Autodesk Fusion 360 part; units mm, degrees
(part 2 of 2)
  spline S394 degree 3 poles (31.1486, 13.7412) (31.2093, 13.8706) (31.3161, 13.9767) (31.4461, 14.036) knots 0.000003 0.000003 0.000003 0.000003 1 1 1 1
  spline S395 degree 3 poles (31.4461, 14.036) (31.5723, 14.0937) (31.7158, 14.1162) (31.8763, 14.1162) knots 0 0 0 0 1 1 1 1
  line L154 (31.8763, 14.1162) -> (34.2237, 14.1162)
  spline S396 degree 3 poles (34.2237, 14.1162) (34.412, 14.1162) (34.5847, 14.0747) (34.7123, 13.9582) knots 0 0 0 0 1 1 1 1
  spline S397 degree 3 poles (34.7123, 13.9582) (34.8291, 13.8516) (34.8932, 13.693) (34.8932, 13.5339) knots 0 0 0 0 1 1 1 1
  spline S398 degree 3 poles (34.8932, 13.5339) (34.8932, 13.3734) (34.8299, 13.2135) (34.7123, 13.1062) knots 0 0 0 0 1 1 1 1
  spline S399 degree 3 poles (34.7123, 13.1062) (34.5847, 12.9897) (34.412, 12.9482) (34.2237, 12.9482) knots 0 0 0 0 1 1 1 1
  line L155 (34.2237, 12.9482) -> (32.4619, 12.9482)
  line L156 (32.4619, 12.9482) -> (32.4619, 12.0907)
  line L157 (32.4619, 12.0907) -> (33.9017, 12.0907)
  spline S400 degree 3 poles (33.9017, 12.0907) (34.0837, 12.0907) (34.2521, 12.0498) (34.3768, 11.9363) knots 0 0 0 0 1 1 1 1
  spline S401 degree 3 poles (34.3768, 11.9363) (34.4927, 11.8307) (34.5545, 11.6729) (34.5545, 11.5151) knots 0 0 0 0 1 1 1 1
  spline S402 degree 3 poles (34.5545, 11.5151) (34.5545, 11.3566) (34.4909, 11.1978) (34.3728, 11.0935) knots 0 0 0 0 1 1 1 1
  spline S403 degree 3 poles (34.3728, 11.0935) (34.2479, 10.9833) (34.0814, 10.9429) (33.9017, 10.9429) knots 0 0 0 0 1 1 1 1
  line L158 (33.9017, 10.9429) -> (32.4619, 10.9429)
  line L159 (32.4619, 10.9429) -> (32.4619, 9.5231)
  spline S404 degree 3 poles (32.4619, 9.5231) (32.4619, 9.2874) (32.4087, 9.0787) (32.269, 8.929) knots 0 0 0 0 1 1 1 1
  spline S405 degree 3 poles (35.2745, 13.3964) (35.2745, 13.628) (35.3278, 13.8341) (35.4642, 13.9838) knots 0 0 0 0 1 1 1 1
  spline S406 degree 3 poles (35.4642, 13.9838) (35.5913, 14.1233) (35.776, 14.2) (35.9675, 14.2) knots 0 0 0 0 1 1 1 1
  spline S407 degree 3 poles (35.9675, 14.2) (36.1615, 14.2) (36.3482, 14.1259) (36.4776, 13.9872) knots 0 0 0 0 1 1 1 1
  spline S408 degree 3 poles (36.4776, 13.9872) (36.6167, 13.838) (36.6705, 13.6302) (36.6705, 13.3964) knots 0 0 0 0 1 1 1 1
  line L160 (36.6705, 13.3964) -> (36.6705, 9.5231)
  spline S409 degree 3 poles (36.6705, 9.5231) (36.6705, 9.2893) (36.6167, 9.0815) (36.4783, 8.9315) knots 0 0 0 0 1 1 1 1
  spline S410 degree 3 poles (36.4783, 8.9315) (36.3492, 8.7914) (36.162, 8.7162) (35.9675, 8.7162) knots 0 0 0 0 1 1 1 1
  spline S411 degree 3 poles (35.9675, 8.7162) (35.777, 8.7162) (35.5932, 8.7944) (35.4659, 8.934) knots 0 0 0 0 1 1 1 1
  spline S412 degree 3 poles (35.4659, 8.934) (35.3289, 9.0842) (35.2745, 9.2912) (35.2745, 9.5231) knots 0 0 0 0 1 1 1 1
  line L161 (35.2745, 9.5231) -> (35.2745, 13.3964)
  spline S413 degree 3 poles (37.4656, 13.7332) (37.4659, 13.7341) (37.4663, 13.7349) (37.4667, 13.7357) (37.5248, 13.8734) (37.6258, 13.9896) (37.7534, 14.0723) knots -0.008376 -0.008376 -0.008376 -0.008376 0 0 0 1 1 1 1
  spline S414 degree 3 poles (37.7534, 14.0723) (37.8814, 14.1552) (38.0295, 14.2) (38.1808, 14.2) knots 0.000001 0.000001 0.000001 0.000001 1 1 1 1
  spline S415 degree 3 poles (38.1808, 14.2) (38.2918, 14.2) (38.3976, 14.1821) (38.4935, 14.1384) knots 0 0 0 0 1 1 1 1
  spline S416 degree 3 poles (38.4935, 14.1384) (38.5787, 14.0995) (38.656, 14.0455) (38.7212, 13.9788) knots 0 0 0 0 1 1 1 1
  spline S417 degree 3 poles (38.7212, 13.9788) (38.7819, 13.9167) (38.8383, 13.8426) (38.8939, 13.756) knots 0 0 0 0 1 1 1 1
  spline S418 degree 3 poles (38.8939, 13.756) (38.9442, 13.6778) (38.9961, 13.5964) (39.0496, 13.5116) knots 0.000001 0.000001 0.000001 0.000001 0.993162 0.993162 0.993162 0.993162
  line L162 (39.0496, 13.5116) -> (40.5964, 11.1711)
  line L163 (40.5964, 11.1711) -> (40.5964, 13.4299)
  spline S419 degree 3 poles (40.5964, 13.4299) (40.5964, 13.6486) (40.6426, 13.8428) (40.7671, 13.9878) knots 0 0 0 0 1 1 1 1
  spline S420 degree 3 poles (40.7671, 13.9878) (40.8852, 14.1253) (41.0649, 14.2) (41.2492, 14.2) knots 0.000007 0.000007 0.000007 0.000007 1 1 1 1
  spline S421 degree 3 poles (41.2492, 14.2) (41.4365, 14.2) (41.6185, 14.1269) (41.7387, 13.9888) knots 0 0 0 0 1 1 1 1
  spline S422 degree 3 poles (41.7387, 13.9888) (41.8648, 13.844) (41.9119, 13.649) (41.9119, 13.4299) knots 0 0 0 0 1 1 1 1
  line L164 (41.9119, 13.4299) -> (41.9119, 9.5634)
  spline S423 degree 3 poles (41.9119, 9.5634) (41.9119, 9.2292) (41.8029, 8.9408) (41.5556, 8.8046) (41.4427, 8.7424) (41.3127, 8.7162) (41.1754, 8.7162) knots 0 0 0 0 0.686484 0.686484 0.686484 1 1 1 1
  spline S424 degree 3 poles (41.1754, 8.7162) (41.0668, 8.7162) (40.9628, 8.7318) (40.8663, 8.7665) knots 0 0 0 0 1 1 1 1
  spline S425 degree 3 poles (40.8663, 8.7665) (40.7688, 8.8015) (40.679, 8.857) (40.5995, 8.9279) knots 0 0 0 0 1 1 1 1
  spline S426 degree 3 poles (40.5995, 8.9279) (40.525, 8.9945) (40.4572, 9.0711) (40.3958, 9.1568) knots 0 0 0 0 1 1 1 1
  spline S427 degree 3 poles (40.3958, 9.1568) (40.3413, 9.2329) (40.2868, 9.3106) (40.2324, 9.3899) (40.232, 9.3905) (40.2316, 9.3912) (40.2311, 9.3918) knots 0 0 0 0 1 1 1 1.008135 1.008135 1.008135 1.008135
  line L165 (40.2311, 9.3918) -> (38.7295, 11.6941)
  line L166 (38.7295, 11.6941) -> (38.7295, 9.4863)
  spline S428 degree 3 poles (38.7295, 9.4863) (38.7295, 9.2675) (38.6776, 9.0701) (38.5469, 8.926) knots 0 0 0 0 1 1 1 1
  spline S429 degree 3 poles (38.5469, 8.926) (38.4248, 8.7914) (38.2467, 8.7162) (38.0634, 8.7162) knots 0.000007 0.000007 0.000007 0.000007 1 1 1 1
  spline S430 degree 3 poles (38.0634, 8.7162) (37.8765, 8.7162) (37.695, 8.792) (37.5741, 8.9305) knots 0 0 0 0 1 1 1 1
  spline S431 degree 3 poles (37.5741, 8.9305) (37.4476, 9.0752) (37.3973, 9.2702) (37.3973, 9.4863) knots 0.000003 0.000003 0.000003 0.000003 1 1 1 1
  line L167 (37.3973, 9.4863) -> (37.3973, 13.279)
  spline S432 degree 3 poles (37.3973, 13.279) (37.3973, 13.4548) (37.4144, 13.6021) (37.4646, 13.7307) (37.4649, 13.7315) (37.4653, 13.7324) (37.4656, 13.7332) knots 0 0 0 0 1 1 1 1.009296 1.009296 1.009296 1.009296
  spline S433 degree 3 poles (9.5214, 6.4924) (9.6235, 6.4007) (9.6809, 6.261) (9.682, 6.1247) knots 0.000001 0.000001 0.000001 0.000001 1 1 1 1
  spline S434 degree 3 poles (9.682, 6.1247) (9.6831, 5.9875) (9.6287, 5.8458) (9.5272, 5.7517) knots 0 0 0 0 1 1 1 1
  spline S435 degree 3 poles (9.5272, 5.7517) (9.4159, 5.6485) (9.267, 5.6129) (9.1105, 5.6116) knots 0.000001 0.000001 0.000001 0.000001 1 1 1 1
  line L168 (9.1105, 5.6116) -> (7.5157, 5.5989)
  line L169 (7.5157, 5.5989) -> (7.5202, 5.0332)
  line L170 (7.5202, 5.0332) -> (8.9728, 5.0447)
  spline S436 degree 3 poles (8.9728, 5.0447) (9.1243, 5.0459) (9.2703, 5.013) (9.3808, 4.914) knots 0 0 0 0 1 1 1 1
  spline S437 degree 3 poles (9.3808, 4.914) (9.4816, 4.8236) (9.5378, 4.6855) (9.5389, 4.5514) knots 0 0 0 0 1 1 1 1
  spline S438 degree 3 poles (9.5389, 4.5514) (9.5399, 4.418) (9.4878, 4.2805) (9.3913, 4.1869) knots 0 0 0 0 1 1 1 1
  spline S439 degree 3 poles (9.3913, 4.1869) (9.2828, 4.0816) (9.1346, 4.045) (8.9807, 4.0438) knots 0 0 0 0 1 1 1 1
  line L171 (8.9807, 4.0438) -> (7.5282, 4.0323)
  line L172 (7.5282, 4.0323) -> (7.5339, 3.3136)
  line L173 (7.5339, 3.3136) -> (9.1903, 3.3267)
  spline S440 degree 3 poles (9.1903, 3.3267) (9.3465, 3.328) (9.4969, 3.2918) (9.6095, 3.1904) knots 0 0 0 0 1 1 1 1
  spline S441 degree 3 poles (9.6095, 3.1904) (9.7144, 3.0958) (9.7716, 2.9525) (9.7727, 2.8121) knots 0.000001 0.000001 0.000001 0.000001 1 1 1 1
  spline S442 degree 3 poles (9.7727, 2.8121) (9.7738, 2.6736) (9.7174, 2.5314) (9.6155, 2.4366) knots 0 0 0 0 1 1 1 1
  spline S443 degree 3 poles (9.6155, 2.4366) (9.5045, 2.3334) (9.3547, 2.2949) (9.1985, 2.2936) knots 0 0 0 0 1 1 1 1
  line L174 (9.1985, 2.2936) -> (7.0336, 2.2764)
  spline S444 degree 3 poles (7.0336, 2.2764) (6.8306, 2.2748) (6.6463, 2.3171) (6.5157, 2.4471) knots 0 0 0 0 1 1 1 1
  spline S445 degree 3 poles (6.5157, 2.4471) (6.3864, 2.5759) (6.3415, 2.758) (6.3399, 2.9592) knots 0 0 0 0 1 1 1 1
  line L175 (6.3399, 2.9592) -> (6.3164, 5.9155)
  spline S446 degree 3 poles (6.3164, 5.9155) (6.3153, 6.0498) (6.3331, 6.1718) (6.3834, 6.2814) knots 0 0 0 0 1 1 1 1
  spline S447 degree 3 poles (6.3834, 6.2814) (6.4347, 6.3931) (6.5275, 6.4867) (6.639, 6.5387) knots 0 0 0 0 1 1 1 1
  spline S448 degree 3 poles (6.639, 6.5387) (6.7467, 6.5889) (6.8669, 6.6082) (6.9992, 6.6092) knots 0.000002 0.000002 0.000002 0.000002 1 1 1 1
  line L176 (6.9992, 6.6092) -> (9.1024, 6.6259)
  spline S449 degree 3 poles (9.1024, 6.6259) (9.259, 6.6272) (9.4084, 6.594) (9.5214, 6.4924) knots 0 0 0 0 1 1 1 1
  spline S450 degree 3 poles (12.5502, 6.0643) (12.5487, 6.2449) (12.5854, 6.4109) (12.6926, 6.5378) knots 0 0 0 0 1 1 1 1
  spline S451 degree 3 poles (12.6926, 6.5378) (12.7934, 6.6571) (12.9505, 6.7236) (13.1071, 6.7248) knots 0 0 0 0 1 1 1 1
  spline S452 degree 3 poles (13.1071, 6.7248) (13.2658, 6.7261) (13.4257, 6.6637) (13.5304, 6.5455) knots 0 0 0 0 1 1 1 1
  spline S453 degree 3 poles (13.5304, 6.5455) (13.6409, 6.4205) (13.6811, 6.2543) (13.6825, 6.0733) knots 0 0 0 0 1 1 1 1
  line L177 (13.6825, 6.0733) -> (13.7071, 2.9802)
  spline S454 degree 3 poles (13.7071, 2.9802) (13.7093, 2.7053) (13.6191, 2.4551) (13.4064, 2.3357) (13.3093, 2.2812) (13.1985, 2.2583) (13.0836, 2.2574) knots 0 0 0 0 0.686484 0.686484 0.686484 1 1 1 1
  spline S455 degree 3 poles (13.0836, 2.2574) (12.9929, 2.2567) (12.9049, 2.2691) (12.8224, 2.298) knots 0 0 0 0 1 1 1 1
  spline S456 degree 3 poles (12.8224, 2.298) (12.739, 2.3272) (12.6623, 2.3739) (12.5948, 2.4331) knots 0 0 0 0 1 1 1 1
  spline S457 degree 3 poles (12.5948, 2.4331) (12.5324, 2.488) (12.4757, 2.5511) (12.4245, 2.6214) knots 0 0 0 0 1 1 1 1
  spline S458 degree 3 poles (12.4245, 2.6214) (12.3802, 2.6821) (12.336, 2.7442) (12.2918, 2.8075) (12.2914, 2.8082) (12.291, 2.8088) (12.2905, 2.8094) knots 0.000004 0.000004 0.000004 0.000004 1 1 1 1.010161 1.010161 1.010161 1.010161
  line L178 (12.2905, 2.8094) -> (11.1488, 4.5299)
  line L179 (11.1488, 4.5299) -> (11.1617, 2.8982)
  spline S459 degree 3 poles (11.1617, 2.8982) (11.1632, 2.7171) (11.1213, 2.5477) (11.009, 2.4219) knots 0 0 0 0 1 1 1 1
  spline S460 degree 3 poles (11.009, 2.4219) (10.9053, 2.3058) (10.7501, 2.2389) (10.594, 2.2376) knots 0 0 0 0 1 1 1 1
  spline S461 degree 3 poles (10.594, 2.2376) (10.4353, 2.2364) (10.2759, 2.3012) (10.171, 2.4194) knots 0 0 0 0 1 1 1 1
  spline S462 degree 3 poles (10.171, 2.4194) (10.0606, 2.5438) (10.0174, 2.7102) (10.016, 2.8891) knots 0 0 0 0 1 1 1 1
  line L180 (10.016, 2.8891) -> (9.9918, 5.9233)
  spline S463 degree 3 poles (9.9918, 5.9233) (9.9907, 6.0668) (10.0033, 6.1889) (10.0455, 6.2996) (10.0458, 6.3004) (10.0461, 6.3013) (10.0464, 6.3021) knots 0 0 0 0 1 1 1 1.011623 1.011623 1.011623 1.011623
  spline S464 degree 3 poles (10.0464, 6.3021) (10.0468, 6.303) (10.0471, 6.3038) (10.0475, 6.3047) (10.0962, 6.4226) (10.1823, 6.523) (10.2897, 6.5938) knots -0.010473 -0.010473 -0.010473 -0.010473 0 0 0 1 1 1 1
  spline S465 degree 3 poles (10.2897, 6.5938) (10.3975, 6.6648) (10.524, 6.7043) (10.6525, 6.7053) knots 0 0 0 0 1 1 1 1
  spline S466 degree 3 poles (10.6525, 6.7053) (10.7457, 6.7061) (10.8362, 6.6918) (10.9196, 6.6545) knots 0 0 0 0 1 1 1 1
  spline S467 degree 3 poles (10.9196, 6.6545) (10.9924, 6.6221) (11.0589, 6.5764) (11.1149, 6.52) knots 0 0 0 0 1 1 1 1
  spline S468 degree 3 poles (11.1149, 6.52) (11.1664, 6.4681) (11.2134, 6.4072) (11.2596, 6.3366) knots 0 0 0 0 1 1 1 1
  spline S469 degree 3 poles (11.2596, 6.3366) (11.3003, 6.2744) (11.3423, 6.2096) (11.3856, 6.1421) knots 0.000001 0.000001 0.000001 0.000001 0.991467 0.991467 0.991467 0.991467
  line L181 (11.3856, 6.1421) -> (12.5635, 4.3904)
  line L182 (12.5635, 4.3904) -> (12.5502, 6.0643)
  spline S470 degree 3 poles (17.5156, 6.1628) (17.5168, 6.0183) (17.4569, 5.8707) (17.349, 5.774) knots 0 0 0 0 1 1 1 1
  spline S471 degree 3 poles (17.349, 5.774) (17.2323, 5.6694) (17.0773, 5.632) (16.912, 5.6307) knots 0.000002 0.000002 0.000002 0.000002 1 1 1 1
  line L183 (16.912, 5.6307) -> (16.2428, 5.6253)
  line L184 (16.2428, 5.6253) -> (16.2639, 2.9683)
  spline S472 degree 3 poles (16.2639, 2.9683) (16.2655, 2.774) (16.2239, 2.5963) (16.105, 2.4653) knots 0 0 0 0 1 1 1 1
  spline S473 degree 3 poles (16.105, 2.4653) (15.997, 2.3461) (15.8369, 2.2793) (15.675, 2.278) knots 0 0 0 0 1 1 1 1
  spline S474 degree 3 poles (15.675, 2.278) (15.5116, 2.2767) (15.3492, 2.3412) (15.2382, 2.4597) knots 0 0 0 0 1 1 1 1
  spline S475 degree 3 poles (15.2382, 2.4597) (15.1174, 2.5886) (15.0714, 2.7657) (15.0699, 2.9588) knots 0 0 0 0 1 1 1 1
  line L185 (15.0699, 2.9588) -> (15.0488, 5.6159)
  line L186 (15.0488, 5.6159) -> (14.3796, 5.6105)
  spline S476 degree 3 poles (14.3796, 5.6105) (14.2143, 5.6092) (14.0586, 5.644) (13.9411, 5.7487) knots 0 0 0 0 1 1 1 1
  spline S477 degree 3 poles (13.9411, 5.7487) (13.8338, 5.8443) (13.7741, 5.9898) (13.773, 6.133) knots 0 0 0 0 1 1 1 1
  spline S478 degree 3 poles (13.773, 6.133) (13.7718, 6.28) (13.8317, 6.4308) (13.943, 6.5277) knots 0 0 0 0 1 1 1 1
  spline S479 degree 3 poles (13.943, 6.5277) (14.0585, 6.6283) (14.2105, 6.6665) (14.3712, 6.6678) knots 0 0 0 0 1 1 1 1
  line L187 (14.3712, 6.6678) -> (16.9036, 6.6879)
  spline S480 degree 3 poles (16.9036, 6.6879) (17.0708, 6.6892) (17.2279, 6.654) (17.3463, 6.5484) knots 0 0 0 0 1 1 1 1
  spline S481 degree 3 poles (17.3463, 6.5484) (17.4539, 6.4524) (17.5145, 6.3066) (17.5156, 6.1628) knots 0 0 0 0 1 1 1 1
  spline S482 degree 3 poles (20.794, 6.582) (20.8961, 6.4902) (20.9535, 6.3505) (20.9546, 6.2142) knots 0.000001 0.000001 0.000001 0.000001 1 1 1 1
  spline S483 degree 3 poles (20.9546, 6.2142) (20.9557, 6.077) (20.9013, 5.9354) (20.7999, 5.8413) knots 0 0 0 0 1 1 1 1
  spline S484 degree 3 poles (20.7999, 5.8413) (20.6885, 5.738) (20.5396, 5.7024) (20.3831, 5.7012) knots 0.000001 0.000001 0.000001 0.000001 1 1 1 1
  line L188 (20.3831, 5.7012) -> (18.7884, 5.6885)
  line L189 (18.7884, 5.6885) -> (18.7929, 5.1227)
  line L190 (18.7929, 5.1227) -> (20.2454, 5.1343)
  spline S485 degree 3 poles (20.2454, 5.1343) (20.3969, 5.1355) (20.5429, 5.1026) (20.6534, 5.0036) knots 0 0 0 0 1 1 1 1
  spline S486 degree 3 poles (20.6534, 5.0036) (20.7542, 4.9132) (20.8104, 4.775) (20.8115, 4.641) knots 0 0 0 0 1 1 1 1
  spline S487 degree 3 poles (20.8115, 4.641) (20.8126, 4.5075) (20.7605, 4.3701) (20.664, 4.2765) knots 0 0 0 0 1 1 1 1
  spline S488 degree 3 poles (20.664, 4.2765) (20.5554, 4.1712) (20.4072, 4.1346) (20.2533, 4.1333) knots 0 0 0 0 1 1 1 1
  line L191 (20.2533, 4.1333) -> (18.8008, 4.1218)
  line L192 (18.8008, 4.1218) -> (18.8065, 3.4031)
  line L193 (18.8065, 3.4031) -> (20.4629, 3.4163)
  spline S489 degree 3 poles (20.4629, 3.4163) (20.6191, 3.4175) (20.7695, 3.3814) (20.8821, 3.2799) knots 0 0 0 0 1 1 1 1
  spline S490 degree 3 poles (20.8821, 3.2799) (20.987, 3.1854) (21.0442, 3.042) (21.0453, 2.9016) knots 0 0 0 0 1 1 1 1
  spline S491 degree 3 poles (21.0453, 2.9016) (21.0464, 2.7631) (20.99, 2.621) (20.8881, 2.5262) knots 0 0 0 0 1 1 1 1
  spline S492 degree 3 poles (20.8881, 2.5262) (20.7771, 2.4229) (20.6273, 2.3844) (20.4711, 2.3832) knots 0 0 0 0 1 1 1 1
  line L194 (20.4711, 2.3832) -> (18.3062, 2.366)
  spline S493 degree 3 poles (18.3062, 2.366) (18.1032, 2.3644) (17.9189, 2.4067) (17.7884, 2.5366) knots 0 0 0 0 1 1 1 1
  spline S494 degree 3 poles (17.7884, 2.5366) (17.659, 2.6654) (17.6141, 2.8476) (17.6125, 3.0488) knots 0 0 0 0 1 1 1 1
  line L195 (17.6125, 3.0488) -> (17.589, 6.0051)
  spline S495 degree 3 poles (17.589, 6.0051) (17.588, 6.1393) (17.6057, 6.2614) (17.656, 6.3709) knots 0 0 0 0 1 1 1 1
  spline S496 degree 3 poles (17.656, 6.3709) (17.7074, 6.4826) (17.8001, 6.5762) (17.9116, 6.6282) knots 0 0 0 0 1 1 1 1
  spline S497 degree 3 poles (17.9116, 6.6282) (18.0193, 6.6784) (18.1395, 6.6977) (18.2718, 6.6988) knots 0 0 0 0 1 1 1 1
  line L196 (18.2718, 6.6988) -> (20.375, 6.7155)
  spline S498 degree 3 poles (20.375, 6.7155) (20.5316, 6.7167) (20.681, 6.6835) (20.794, 6.582) knots 0 0 0 0 1 1 1 1
  spline S499 degree 3 poles (24.0991, 4.3138) (24.1406, 4.2747) (24.1812, 4.2328) (24.2209, 4.1883) knots 0.721867 0.721867 0.721867 0.721867 1 1 1 1
  spline S500 degree 3 poles (24.2209, 4.1883) (24.3584, 4.0342) (24.4815, 3.8698) (24.5899, 3.6954) knots 0 0 0 0 1 1 1 1
  spline S501 degree 3 poles (24.5899, 3.6954) (24.6962, 3.5245) (24.7807, 3.3679) (24.8433, 3.223) knots 0 0 0 0 1 1 1 1
  spline S502 degree 3 poles (24.8433, 3.223) (24.9043, 3.0819) (24.9454, 2.996) (24.9464, 2.8709) knots 0.000002 0.000002 0.000002 0.000002 1 1 1 1
  spline S503 degree 3 poles (24.9464, 2.8709) (24.9472, 2.7765) (24.916, 2.6845) (24.8666, 2.6071) knots 0 0 0 0 1 1 1 1
  spline S504 degree 3 poles (24.8666, 2.6071) (24.8151, 2.5264) (24.7412, 2.4603) (24.6566, 2.4159) knots 0.00001 0.00001 0.00001 0.00001 1 1 1 1
  spline S505 degree 3 poles (24.6566, 2.4159) (24.568, 2.3693) (24.4682, 2.3479) (24.3669, 2.3471) knots 0 0 0 0 1 1 1 1
  spline S506 degree 3 poles (24.3669, 2.3471) (24.2462, 2.3461) (24.1261, 2.3756) (24.0271, 2.4429) knots 0 0 0 0 1 1 1 1
  spline S507 degree 3 poles (24.0271, 2.4429) (23.945, 2.4986) (23.8741, 2.5701) (23.8168, 2.6528) knots 0 0 0 0 1 1 1 1
  spline S508 degree 3 poles (23.8168, 2.6528) (23.7684, 2.7227) (23.7071, 2.819) (23.6299, 2.9454) knots 0 0 0 0 1 1 1 1
  line L197 (23.6299, 2.9454) -> (23.306, 3.4747)
  spline S509 degree 3 poles (23.306, 3.4747) (23.3059, 3.475) (23.3057, 3.4753) (23.3055, 3.4756) (23.1935, 3.663) (23.0947, 3.802) (23.0178, 3.8873) knots -0.00151 -0.00151 -0.00151 -0.00151 0 0 0 1 1 1 1
  spline S510 degree 3 poles (23.0178, 3.8873) (22.9413, 3.9723) (22.8722, 4.0202) (22.8164, 4.0422) knots 0.000003 0.000003 0.000003 0.000003 1 1 1 1
  spline S511 degree 3 poles (22.8164, 4.0422) (22.7558, 4.0661) (22.6631, 4.0827) (22.5395, 4.0818) knots 0 0 0 0 1 1 1 1
  line L198 (22.5395, 4.0818) -> (22.4605, 4.0811)
  line L199 (22.4605, 4.0811) -> (22.469, 3.0176)
  spline S512 degree 3 poles (22.469, 3.0176) (22.4705, 2.8219) (22.4295, 2.6435) (22.3093, 2.5124) knots 0 0 0 0 1 1 1 1
  spline S513 degree 3 poles (22.3093, 2.5124) (22.2004, 2.3937) (22.0399, 2.3286) (21.8774, 2.3273) knots 0 0 0 0 1 1 1 1
  spline S514 degree 3 poles (21.8774, 2.3273) (21.7072, 2.3259) (21.5377, 2.3907) (21.4282, 2.5178) knots 0 0 0 0 1 1 1 1
  spline S515 degree 3 poles (21.4282, 2.5178) (21.3163, 2.6477) (21.2737, 2.8197) (21.2722, 3.0081) knots 0.000001 0.000001 0.000001 0.000001 1 1 1 1
  line L200 (21.2722, 3.0081) -> (21.2482, 6.0341)
  spline S516 degree 3 poles (21.2482, 6.0341) (21.2466, 6.2357) (21.2895, 6.4193) (21.418, 6.5498) knots 0 0 0 0 1 1 1 1
  spline S517 degree 3 poles (21.418, 6.5498) (21.5465, 6.6804) (21.7294, 6.7262) (21.931, 6.7278) knots 0 0 0 0 1 1 1 1
  line L201 (21.931, 6.7278) -> (23.2267, 6.7381)
  spline S518 degree 3 poles (23.2267, 6.7381) (23.4112, 6.7396) (23.5713, 6.7332) (23.7094, 6.7177) knots 0 0 0 0 1 1 1 1
  spline S519 degree 3 poles (23.7094, 6.7177) (23.8531, 6.7017) (23.9874, 6.6674) (24.1101, 6.613) knots 0 0 0 0 0.992566 0.992566 0.992566 0.992566
  spline S520 degree 3 poles (24.1101, 6.613) (24.2569, 6.5522) (24.3892, 6.4635) (24.502, 6.3503) knots 0.006255 0.006255 0.006255 0.006255 1 1 1 1
  spline S521 degree 3 poles (24.502, 6.3503) (24.6165, 6.2355) (24.7053, 6.0993) (24.7651, 5.9474) knots 0 0 0 0 1 1 1 1
  spline S522 degree 3 poles (24.7651, 5.9474) (24.8245, 5.7967) (24.8547, 5.6359) (24.856, 5.4699) knots 0 0 0 0 1 1 1 1
  spline S523 degree 3 poles (24.856, 5.4699) (24.8586, 5.139) (24.7619, 4.8447) (24.56, 4.6273) knots 0 0 0 0 1 1 1 1
  spline S524 degree 3 poles (24.56, 4.6273) (24.4382, 4.4963) (24.2827, 4.3929) (24.0991, 4.3138) knots 0 0 0 0 0.606921 0.606921 0.606921 0.606921
  spline S525 degree 3 poles (27.0403, 3.0539) (27.0418, 2.8596) (27.0002, 2.6819) (26.8813, 2.5509) knots 0 0 0 0 1 1 1 1
  spline S526 degree 3 poles (26.8813, 2.5509) (26.7733, 2.4317) (26.6133, 2.3649) (26.4514, 2.3636) knots 0.000003 0.000003 0.000003 0.000003 1 1 1 1
  spline S527 degree 3 poles (26.4514, 2.3636) (26.2879, 2.3623) (26.1255, 2.4268) (26.0145, 2.5453) knots 0 0 0 0 1 1 1 1
  spline S528 degree 3 poles (26.0145, 2.5453) (25.8937, 2.6742) (25.8477, 2.8513) (25.8462, 3.0444) knots 0.000001 0.000001 0.000001 0.000001 1 1 1 1
  line L202 (25.8462, 3.0444) -> (25.8251, 5.7015)
  line L203 (25.8251, 5.7015) -> (25.1559, 5.6962)
  spline S529 degree 3 poles (25.1559, 5.6962) (24.9906, 5.6948) (24.8349, 5.7296) (24.7174, 5.8343) knots 0 0 0 0 1 1 1 1
  spline S530 degree 3 poles (24.7174, 5.8343) (24.6101, 5.9299) (24.5505, 6.0754) (24.5493, 6.2186) knots 0 0 0 0 1 1 1 1
  spline S531 degree 3 poles (24.5493, 6.2186) (24.5482, 6.3656) (24.608, 6.5164) (24.7193, 6.6133) knots 0 0 0 0 1 1 1 1
  spline S532 degree 3 poles (24.7193, 6.6133) (24.8348, 6.7139) (24.9868, 6.7521) (25.1475, 6.7534) knots 0 0 0 0 1 1 1 1
  line L204 (25.1475, 6.7534) -> (27.68, 6.7735)
  spline S533 degree 3 poles (27.68, 6.7735) (27.8471, 6.7748) (28.0042, 6.7396) (28.1226, 6.634) knots 0 0 0 0 1 1 1 1
  spline S534 degree 3 poles (28.1226, 6.634) (28.2302, 6.538) (28.2908, 6.3922) (28.2919, 6.2484) knots 0.000005 0.000005 0.000005 0.000005 1 1 1 1
  spline S535 degree 3 poles (28.2919, 6.2484) (28.2931, 6.104) (28.2332, 5.9563) (28.1253, 5.8596) knots 0 0 0 0 1 1 1 1
  spline S536 degree 3 poles (28.1253, 5.8596) (28.0086, 5.755) (27.8537, 5.7176) (27.6883, 5.7163) knots 0 0 0 0 1 1 1 1
  line L205 (27.6883, 5.7163) -> (27.0192, 5.711)
  line L206 (27.0192, 5.711) -> (27.0403, 3.0539)
  spline S537 degree 3 poles (31.811, 2.9711) (31.8122, 2.8243) (31.745, 2.6826) (31.6416, 2.5774) knots 0 0 0 0 1 1 1 1
  spline S538 degree 3 poles (31.6415, 2.5774) (31.5331, 2.4673) (31.3811, 2.4028) (31.2265, 2.4015) knots 0 0 0 0 1 1 1 1
  spline S539 degree 3 poles (31.2265, 2.4015) (31.1401, 2.4009) (31.0541, 2.4158) (30.9757, 2.4542) knots 0 0 0 0 1 1 1 1
  spline S540 degree 3 poles (30.9757, 2.4542) (30.9059, 2.4884) (30.8432, 2.5381) (30.7944, 2.5988) knots 0.000006 0.000006 0.000006 0.000006 1 1 1 1
  spline S541 degree 3 poles (30.7944, 2.5988) (30.745, 2.6604) (30.7079, 2.7307) (30.6685, 2.8187) knots 0 0 0 0 1 1 1 1
  spline S542 degree 3 poles (30.6685, 2.8187) (30.6325, 2.899) (30.6014, 2.9702) (30.5751, 3.0326) (30.5748, 3.0335) (30.5744, 3.0343) (30.5741, 3.0351) knots 0.000001 0.000001 0.000001 0.000001 1 1 1 1.013735 1.013735 1.013735 1.013735
  line L207 (30.5741, 3.0351) -> (30.4314, 3.4013)
  line L208 (30.4314, 3.4013) -> (29.1094, 3.3908)
  line L209 (29.1094, 3.3908) -> (28.9731, 3.0156)
  spline S543 degree 3 poles (28.9731, 3.0156) (28.9731, 3.0156) (28.9731, 3.0155) (28.973, 3.0155) (28.8986, 2.8109) (28.84, 2.6713) (28.7612, 2.5649) knots -0.000204 -0.000204 -0.000204 -0.000204 0 0 0 1 1 1 1
  spline S544 degree 3 poles (28.7612, 2.5649) (28.6664, 2.4371) (28.5049, 2.3799) (28.348, 2.3787) knots 0.000001 0.000001 0.000001 0.000001 1 1 1 1
  spline S545 degree 3 poles (28.348, 2.3787) (28.1991, 2.3775) (28.0522, 2.4383) (27.9431, 2.5407) knots 0 0 0 0 1 1 1 1
  spline S546 degree 3 poles (27.9431, 2.5407) (27.8348, 2.6423) (27.7638, 2.7854) (27.7626, 2.9335) knots 0 0 0 0 1 1 1 1
  spline S547 degree 3 poles (27.7626, 2.9335) (27.762, 3.0094) (27.7742, 3.0854) (27.7968, 3.1598) knots 0 0 0 0 1 1 1 1
  spline S548 degree 3 poles (27.7968, 3.1598) (27.8171, 3.2266) (27.8473, 3.3095) (27.8887, 3.4145) knots 0 0 0 0 1 1 1 1
  line L210 (27.8887, 3.4145) -> (28.8736, 5.9743)
  spline S549 degree 3 poles (28.8736, 5.9743) (28.9017, 6.0479) (28.9354, 6.1363) (28.9748, 6.2395) knots 0 0 0 0 1 1 1 1
  spline S550 degree 3 poles (28.9748, 6.2395) (29.0181, 6.3526) (29.0657, 6.4509) (29.1215, 6.5354) knots 0.000007 0.000007 0.000007 0.000007 1 1 1 1
  spline S551 degree 3 poles (29.1215, 6.5354) (29.1837, 6.6297) (29.2682, 6.708) (29.3669, 6.765) knots 0.000009 0.000009 0.000009 0.000009 1 1 1 1
  spline S552 degree 3 poles (29.3669, 6.765) (29.4772, 6.8286) (29.6049, 6.8559) (29.7397, 6.8569) knots 0 0 0 0 1 1 1 1
  spline S553 degree 3 poles (29.7397, 6.8569) (29.8759, 6.858) (30.0047, 6.8331) (30.1166, 6.7709) knots 0 0 0 0 1 1 1 1
  spline S554 degree 3 poles (30.1166, 6.7709) (30.2152, 6.7162) (30.3004, 6.6412) (30.3643, 6.55) knots 0 0 0 0 1 1 1 1
  spline S555 degree 3 poles (30.3643, 6.55) (30.4187, 6.4724) (30.4646, 6.389) (30.5019, 6.3005) knots 0 0 0 0 1 1 1 1
  spline S556 degree 3 poles (30.5019, 6.3005) (30.5348, 6.2224) (30.5756, 6.1206) (30.6249, 5.9939) knots 0 0 0 0 0.994802 0.994802 0.994802 0.994802
  line L211 (30.6249, 5.9939) -> (31.6717, 3.4662)
  spline S557 degree 3 poles (31.6718, 3.4662) (31.7575, 3.2648) (31.8098, 3.1195) (31.811, 2.9711) knots 0.003062 0.003062 0.003062 0.003062 1 1 1 1
  spline S558 degree 3 poles (32.1607, 6.6901) (32.2685, 6.8104) (32.429, 6.8783) (32.5914, 6.8796) knots 0.000004 0.000004 0.000004 0.000004 1 1 1 1
  spline S559 degree 3 poles (32.5914, 6.8796) (32.7555, 6.8809) (32.9184, 6.8181) (33.0302, 6.7001) knots 0 0 0 0 1 1 1 1
  spline S560 degree 3 poles (33.0302, 6.7001) (33.1518, 6.5717) (33.1977, 6.3947) (33.1992, 6.2015) knots 0 0 0 0 1 1 1 1
  line L212 (33.1992, 6.2015) -> (33.2238, 3.103)
  spline S561 degree 3 poles (33.2238, 3.103) (33.2254, 2.9099) (33.1822, 2.7321) (33.0635, 2.6013) knots 0 0 0 0 1 1 1 1
  spline S562 degree 3 poles (33.0635, 2.6013) (32.9539, 2.4805) (32.7915, 2.414) (32.6269, 2.4127) knots 0.000001 0.000001 0.000001 0.000001 1 1 1 1
  spline S563 degree 3 poles (32.6269, 2.4127) (32.465, 2.4114) (32.3043, 2.4782) (32.1946, 2.5965) knots 0 0 0 0 1 1 1 1
  spline S564 degree 3 poles (32.1946, 2.5965) (32.0751, 2.7255) (32.0286, 2.9018) (32.0271, 3.0935) knots 0 0 0 0 1 1 1 1
  line L213 (32.0271, 3.0935) -> (32.0025, 6.192)
  spline S565 degree 3 poles (32.0025, 6.192) (32.001, 6.3833) (32.0437, 6.5597) (32.1607, 6.6901) knots 0 0 0 0 1 1 1 1
  spline S566 degree 3 poles (33.756, 6.4905) (33.7563, 6.4913) (33.7567, 6.4922) (33.757, 6.493) (33.8057, 6.6109) (33.8918, 6.7114) (33.9993, 6.7822) knots -0.010469 -0.010469 -0.010469 -0.010469 0 0 0 1 1 1 1
  spline S567 degree 3 poles (33.9993, 6.7822) (34.107, 6.8532) (34.2335, 6.8926) (34.362, 6.8937) knots 0 0 0 0 1 1 1 1
  spline S568 degree 3 poles (34.362, 6.8937) (34.4552, 6.8944) (34.5457, 6.8801) (34.6292, 6.8429) knots 0 0 0 0 1 1 1 1
  spline S569 degree 3 poles (34.6292, 6.8429) (34.7019, 6.8104) (34.7684, 6.7648) (34.8244, 6.7083) knots 0 0 0 0 1 1 1 1
  spline S570 degree 3 poles (34.8244, 6.7083) (34.876, 6.6564) (34.9229, 6.5955) (34.9691, 6.5249) knots 0.000017 0.000017 0.000017 0.000017 1 1 1 1
  spline S571 degree 3 poles (34.9691, 6.5249) (35.0098, 6.4627) (35.0518, 6.3979) (35.0952, 6.3305) knots 0 0 0 0 0.991468 0.991468 0.991468 0.991468
  line L214 (35.0952, 6.3305) -> (36.273, 4.5787)
  line L215 (36.273, 4.5787) -> (36.2597, 6.2526)
  spline S572 degree 3 poles (36.2597, 6.2526) (36.2582, 6.4333) (36.2949, 6.5993) (36.4021, 6.7262) knots 0 0 0 0 1 1 1 1
  spline S573 degree 3 poles (36.4021, 6.7262) (36.5029, 6.8454) (36.66, 6.9119) (36.8166, 6.9132) knots 0 0 0 0 1 1 1 1
  spline S574 degree 3 poles (36.8166, 6.9132) (36.9754, 6.9144) (37.1352, 6.8521) (37.2399, 6.7338) knots 0 0 0 0 1 1 1 1
  spline S575 degree 3 poles (37.2399, 6.7338) (37.3504, 6.6089) (37.3906, 6.4427) (37.392, 6.2616) knots 0 0 0 0 1 1 1 1
  line L216 (37.392, 6.2616) -> (37.4166, 3.1685)
  spline S576 degree 3 poles (37.4166, 3.1685) (37.4188, 2.8936) (37.3286, 2.6434) (37.1159, 2.5241) (37.0188, 2.4695) (36.908, 2.4467) (36.7931, 2.4458) knots 0 0 0 0 0.686484 0.686484 0.686484 1 1 1 1
  spline S577 degree 3 poles (36.7931, 2.4458) (36.7024, 2.445) (36.6144, 2.4574) (36.532, 2.4863) knots 0 0 0 0 1 1 1 1
  spline S578 degree 3 poles (36.532, 2.4863) (36.4486, 2.5156) (36.3718, 2.5622) (36.3043, 2.6215) knots 0 0 0 0 1 1 1 1
  spline S579 degree 3 poles (36.3043, 2.6215) (36.2419, 2.6763) (36.1852, 2.7395) (36.134, 2.8098) knots 0 0 0 0 1 1 1 1
  spline S580 degree 3 poles (36.134, 2.8098) (36.0897, 2.8705) (36.0455, 2.9325) (36.0013, 2.9959) (36.0009, 2.9965) (36.0005, 2.9971) (36, 2.9978) knots 0 0 0 0 1 1 1 1.010164 1.010164 1.010164 1.010164
  line L217 (36, 2.9978) -> (34.8583, 4.7183)
  line L218 (34.8583, 4.7183) -> (34.8712, 3.0866)
  spline S581 degree 3 poles (34.8712, 3.0866) (34.8727, 2.9054) (34.8308, 2.7361) (34.7185, 2.6103) knots 0 0 0 0 1 1 1 1
  spline S582 degree 3 poles (34.7185, 2.6103) (34.6148, 2.4941) (34.4597, 2.4272) (34.3036, 2.426) knots 0 0 0 0 1 1 1 1
  spline S583 degree 3 poles (34.3036, 2.426) (34.1449, 2.4247) (33.9855, 2.4895) (33.8805, 2.6078) knots 0 0 0 0 1 1 1 1
  spline S584 degree 3 poles (33.8805, 2.6078) (33.7701, 2.7321) (33.7269, 2.8985) (33.7255, 3.0775) knots 0 0 0 0 1 1 1 1
  line L219 (33.7255, 3.0775) -> (33.7014, 6.1116)
  spline S585 degree 3 poles (33.7014, 6.1116) (33.7002, 6.2552) (33.7128, 6.3773) (33.755, 6.4879) (33.7553, 6.4888) (33.7556, 6.4896) (33.756, 6.4905) knots 0 0 0 0 1 1 1 1.011619 1.011619 1.011619 1.011619
  spline S586 degree 3 poles (38.0482, 6.7322) (38.1804, 6.8223) (38.3424, 6.8582) (38.5207, 6.8596) knots 0.000003 0.000003 0.000003 0.000003 1 1 1 1
  line L220 (38.5207, 6.8596) -> (38.7675, 6.8616)
  spline S587 degree 3 poles (38.7675, 6.8616) (38.928, 6.8629) (39.0508, 6.855) (39.1654, 6.8102) knots 0 0 0 0 1 1 1 1
  spline S588 degree 3 poles (39.1654, 6.8102) (39.2781, 6.7662) (39.3725, 6.674) (39.4236, 6.5655) knots 0.000001 0.000001 0.000001 0.000001 1 1 1 1
  spline S589 degree 3 poles (39.4236, 6.5655) (39.4669, 6.4735) (39.5046, 6.3549) (39.5485, 6.1925) knots 0.000001 0.000001 0.000001 0.000001 1 1 1 1
  line L221 (39.5485, 6.1925) -> (39.9377, 4.7708)
  line L222 (39.9377, 4.7708) -> (40.3043, 6.1985)
  spline S590 degree 3 poles (40.3043, 6.1985) (40.3455, 6.3616) (40.3814, 6.4808) (40.4232, 6.5734) knots 0 0 0 0 1 1 1 1
  spline S591 degree 3 poles (40.4232, 6.5734) (40.4726, 6.6827) (40.5655, 6.7764) (40.6775, 6.8222) knots 0.000001 0.000001 0.000001 0.000001 1 1 1 1
  spline S592 degree 3 poles (40.6775, 6.8222) (40.7914, 6.8688) (40.9141, 6.8786) (41.0746, 6.8799) knots 0.000006 0.000006 0.000006 0.000006 1 1 1 1
  line L223 (41.0746, 6.8799) -> (41.3214, 6.8819)
  spline S593 degree 3 poles (41.3214, 6.8819) (41.4997, 6.8833) (41.6622, 6.85) (41.7958, 6.7619) knots 0 0 0 0 1 1 1 1
  spline S594 degree 3 poles (41.7958, 6.7619) (41.9595, 6.6541) (42.0211, 6.4566) (42.0227, 6.2501) knots 0 0 0 0 1 1 1 1
  line L224 (42.0227, 6.2501) -> (42.0474, 3.1382)
  spline S595 degree 3 poles (42.0474, 3.1382) (42.0489, 2.9582) (42.01, 2.7912) (41.8998, 2.6658) knots 0 0 0 0 1 1 1 1
  spline S596 degree 3 poles (41.8998, 2.6658) (41.7966, 2.5484) (41.6395, 2.4843) (41.4824, 2.483) knots 0.000005 0.000005 0.000005 0.000005 1 1 1 1
  spline S597 degree 3 poles (41.4824, 2.483) (41.3294, 2.4818) (41.1759, 2.5458) (41.0725, 2.6583) knots 0 0 0 0 1 1 1 1
  spline S598 degree 3 poles (41.0725, 2.6583) (40.959, 2.7817) (40.9165, 2.9488) (40.9151, 3.1292) knots 0 0 0 0 1 1 1 1
  line L225 (40.9151, 3.1292) -> (40.9063, 4.2296)
  line L226 (40.9063, 4.2296) -> (40.6774, 3.288)
  spline S599 degree 3 poles (40.6774, 3.288) (40.6773, 3.2879) (40.6773, 3.2877) (40.6773, 3.2876) (40.6368, 3.122) (40.6039, 3) (40.575, 2.9131) knots -0.000844 -0.000844 -0.000844 -0.000844 0 0 0 1 1 1 1
  spline S600 degree 3 poles (40.575, 2.9131) (40.5377, 2.8008) (40.468, 2.7013) (40.3781, 2.6193) knots 0 0 0 0 1 1 1 1
  spline S601 degree 3 poles (40.3781, 2.6193) (40.2655, 2.5166) (40.1132, 2.4721) (39.956, 2.4709) knots 0 0 0 0 1 1 1 1
  spline S602 degree 3 poles (39.956, 2.4709) (39.8341, 2.4699) (39.7148, 2.4966) (39.6132, 2.5589) knots 0 0 0 0 1 1 1 1
  spline S603 degree 3 poles (39.6132, 2.5589) (39.5229, 2.6143) (39.4465, 2.6908) (39.3935, 2.7818) knots 0.000007 0.000007 0.000007 0.000007 1 1 1 1
  spline S604 degree 3 poles (39.3935, 2.7818) (39.348, 2.86) (39.3129, 2.9452) (39.2876, 3.0359) knots 0.000013 0.000013 0.000013 0.000013 1 1 1 1
  spline S605 degree 3 poles (39.2876, 3.0359) (39.2662, 3.1124) (39.2444, 3.1919) (39.2222, 3.2746) (39.2221, 3.2748) (39.222, 3.2751) (39.2219, 3.2754) knots 0 0 0 0 1 1 1 1.003409 1.003409 1.003409 1.003409
  line L227 (39.2219, 3.2754) -> (38.9778, 4.2143)
  line L228 (38.9778, 4.2143) -> (38.9865, 3.1139)
  spline S606 degree 3 poles (38.9865, 3.1139) (38.9879, 2.9339) (38.949, 2.7669) (38.8388, 2.6415) knots 0 0 0 0 1 1 1 1
  spline S607 degree 3 poles (38.8388, 2.6415) (38.7362, 2.5247) (38.5802, 2.46) (38.4242, 2.4587) knots 0 0 0 0 1 1 1 1
  spline S608 degree 3 poles (38.4242, 2.4587) (38.2707, 2.4575) (38.1166, 2.5197) (38.0124, 2.6317) knots 0 0 0 0 1 1 1 1
  spline S609 degree 3 poles (38.0124, 2.6317) (37.8975, 2.7552) (37.8556, 2.9231) (37.8541, 3.1049) knots 0 0 0 0 1 1 1 1
  line L229 (37.8541, 3.1049) -> (37.8294, 6.2168)
  spline S610 degree 3 poles (37.8294, 6.2168) (37.8278, 6.4232) (37.8862, 6.6218) (38.0482, 6.7322) knots 0 0 0 0 1 1 1 1
  spline S611 degree 3 poles (45.6463, 6.7794) (45.7484, 6.6877) (45.8059, 6.548) (45.8069, 6.4117) knots 0 0 0 0 1 1 1 1
  spline S612 degree 3 poles (45.8069, 6.4117) (45.808, 6.2744) (45.7536, 6.1328) (45.6522, 6.0387) knots 0 0 0 0 1 1 1 1
  spline S613 degree 3 poles (45.6522, 6.0387) (45.5409, 5.9354) (45.392, 5.8998) (45.2354, 5.8986) knots 0 0 0 0 1 1 1 1
  line L230 (45.2354, 5.8986) -> (43.6407, 5.8859)
  line L231 (43.6407, 5.8859) -> (43.6452, 5.3201)
  line L232 (43.6452, 5.3201) -> (45.0977, 5.3317)
  spline S614 degree 3 poles (45.0977, 5.3317) (45.2492, 5.3329) (45.3952, 5.3) (45.5057, 5.201) knots 0 0 0 0 1 1 1 1
  spline S615 degree 3 poles (45.5057, 5.201) (45.6066, 5.1106) (45.6628, 4.9725) (45.6638, 4.8384) knots 0.000006 0.000006 0.000006 0.000006 1 1 1 1
  spline S616 degree 3 poles (45.6638, 4.8384) (45.6649, 4.705) (45.6128, 4.5675) (45.5163, 4.4739) knots 0 0 0 0 1 1 1 1
  spline S617 degree 3 poles (45.5163, 4.4739) (45.4077, 4.3686) (45.2595, 4.332) (45.1057, 4.3308) knots 0 0 0 0 1 1 1 1
  line L233 (45.1057, 4.3308) -> (43.6531, 4.3192)
  line L234 (43.6531, 4.3192) -> (43.6588, 3.6005)
  line L235 (43.6588, 3.6005) -> (45.3153, 3.6137)
  spline S618 degree 3 poles (45.3153, 3.6137) (45.4714, 3.6149) (45.6219, 3.5788) (45.7344, 3.4774) knots 0 0 0 0 1 1 1 1
  spline S619 degree 3 poles (45.7344, 3.4774) (45.8394, 3.3828) (45.8965, 3.2395) (45.8976, 3.0991) knots 0.000001 0.000001 0.000001 0.000001 1 1 1 1
  spline S620 degree 3 poles (45.8976, 3.0991) (45.8987, 2.9606) (45.8424, 2.8184) (45.7404, 2.7236) knots 0 0 0 0 1 1 1 1
  spline S621 degree 3 poles (45.7404, 2.7236) (45.6295, 2.6204) (45.4796, 2.5818) (45.3235, 2.5806) knots 0 0 0 0 1 1 1 1
  line L236 (45.3235, 2.5806) -> (43.1586, 2.5634)
  spline S622 degree 3 poles (43.1586, 2.5634) (42.9555, 2.5618) (42.7712, 2.6041) (42.6407, 2.7341) knots 0 0 0 0 1 1 1 1
  spline S623 degree 3 poles (42.6407, 2.7341) (42.5113, 2.8629) (42.4664, 3.045) (42.4648, 3.2462) knots 0 0 0 0 1 1 1 1
  line L237 (42.4648, 3.2462) -> (42.4414, 6.2025)
  spline S624 degree 3 poles (42.4414, 6.2025) (42.4403, 6.3367) (42.458, 6.4588) (42.5084, 6.5683) knots 0 0 0 0 1 1 1 1
  spline S625 degree 3 poles (42.5084, 6.5683) (42.5597, 6.68) (42.6525, 6.7736) (42.7639, 6.8256) knots 0 0 0 0 1 1 1 1
  spline S626 degree 3 poles (42.7639, 6.8256) (42.8716, 6.8759) (42.9919, 6.8951) (43.1241, 6.8962) knots 0.000001 0.000001 0.000001 0.000001 1 1 1 1
  line L238 (43.1241, 6.8962) -> (45.2274, 6.9129)
  spline S627 degree 3 poles (45.2274, 6.9129) (45.3839, 6.9141) (45.5333, 6.8809) (45.6463, 6.7794) knots 0 0 0 0 1 1 1 1
  spline S628 degree 3 poles (48.6751, 6.3513) (48.6737, 6.5319) (48.7103, 6.6979) (48.8176, 6.8248) knots 0 0 0 0 1 1 1 1
  spline S629 degree 3 poles (48.8176, 6.8248) (48.9184, 6.9441) (49.0755, 7.0105) (49.2321, 7.0118) knots 0 0 0 0 1 1 1 1
  spline S630 degree 3 poles (49.2321, 7.0118) (49.3908, 7.0131) (49.5507, 6.9507) (49.6553, 6.8325) knots 0 0 0 0 1 1 1 1
  spline S631 degree 3 poles (49.6553, 6.8325) (49.7658, 6.7075) (49.806, 6.5413) (49.8075, 6.3603) knots 0.000005 0.000005 0.000005 0.000005 1 1 1 1
  line L239 (49.8075, 6.3603) -> (49.832, 3.2671)
  spline S632 degree 3 poles (49.832, 3.2671) (49.8342, 2.9922) (49.744, 2.742) (49.5314, 2.6227) (49.4343, 2.5682) (49.3234, 2.5453) (49.2085, 2.5444) knots 0 0 0 0 0.686484 0.686484 0.686484 1 1 1 1
  spline S633 degree 3 poles (49.2085, 2.5444) (49.1178, 2.5437) (49.0298, 2.5561) (48.9474, 2.585) knots 0 0 0 0 1 1 1 1
  spline S634 degree 3 poles (48.9474, 2.585) (48.864, 2.6142) (48.7872, 2.6609) (48.7198, 2.7201) knots 0 0 0 0 1 1 1 1
  spline S635 degree 3 poles (48.7198, 2.7201) (48.6573, 2.775) (48.6006, 2.8381) (48.5494, 2.9084) knots 0 0 0 0 1 1 1 1
  spline S636 degree 3 poles (48.5494, 2.9084) (48.5052, 2.9691) (48.461, 3.0312) (48.4168, 3.0945) (48.4163, 3.0951) (48.4159, 3.0958) (48.4155, 3.0964) knots 0 0 0 0 1 1 1 1.010149 1.010149 1.010149 1.010149
  line L240 (48.4155, 3.0964) -> (47.2737, 4.8169)
  line L241 (47.2737, 4.8169) -> (47.2867, 3.1852)
  spline S637 degree 3 poles (47.2867, 3.1852) (47.2881, 3.004) (47.2463, 2.8347) (47.134, 2.7089) knots 0 0 0 0 1 1 1 1
  spline S638 degree 3 poles (47.134, 2.7089) (47.0303, 2.5927) (46.8751, 2.5259) (46.719, 2.5246) knots 0 0 0 0 1 1 1 1
  spline S639 degree 3 poles (46.719, 2.5246) (46.5603, 2.5234) (46.4009, 2.5882) (46.296, 2.7064) knots 0 0 0 0 1 1 1 1
  spline S640 degree 3 poles (46.296, 2.7064) (46.1855, 2.8308) (46.1423, 2.9972) (46.1409, 3.1761) knots 0 0 0 0 1 1 1 1
  line L242 (46.1409, 3.1761) -> (46.1168, 6.2102)
  spline S641 degree 3 poles (46.1168, 6.2102) (46.1157, 6.3538) (46.1283, 6.4759) (46.1704, 6.5865) (46.1707, 6.5874) (46.1711, 6.5882) (46.1714, 6.5891) knots 0 0 0 0 1 1 1 1.011626 1.011626 1.011626 1.011626
  spline S642 degree 3 poles (46.1714, 6.5891) (46.1717, 6.5899) (46.1721, 6.5908) (46.1724, 6.5916) (46.2211, 6.7095) (46.3073, 6.81) (46.4147, 6.8808) knots -0.010475 -0.010475 -0.010475 -0.010475 0 0 0 1 1 1 1
  spline S643 degree 3 poles (46.4147, 6.8808) (46.5224, 6.9518) (46.6489, 6.9913) (46.7774, 6.9923) knots 0 0 0 0 1 1 1 1
  spline S644 degree 3 poles (46.7774, 6.9923) (46.8706, 6.993) (46.9612, 6.9788) (47.0446, 6.9415) knots 0 0 0 0 1 1 1 1
  spline S645 degree 3 poles (47.0446, 6.9415) (47.1173, 6.909) (47.1838, 6.8634) (47.2398, 6.807) knots 0.000017 0.000017 0.000017 0.000017 1 1 1 1
  spline S646 degree 3 poles (47.2398, 6.807) (47.2914, 6.7551) (47.3384, 6.6941) (47.3845, 6.6236) knots 0 0 0 0 1 1 1 1
  spline S647 degree 3 poles (47.3845, 6.6236) (47.4252, 6.5613) (47.4673, 6.4965) (47.5106, 6.4291) knots 0 0 0 0 0.991469 0.991469 0.991469 0.991469
  line L243 (47.5106, 6.4291) -> (48.6884, 4.6773)
  line L244 (48.6884, 4.6773) -> (48.6751, 6.3513)
  spline S648 degree 3 poles (53.4712, 6.8353) (53.5788, 6.7393) (53.6394, 6.5936) (53.6405, 6.4497) knots 0 0 0 0 1 1 1 1
  spline S649 degree 3 poles (53.6405, 6.4497) (53.6417, 6.3053) (53.5819, 6.1576) (53.4739, 6.061) knots 0 0 0 0 1 1 1 1
  spline S650 degree 3 poles (53.4739, 6.061) (53.3572, 5.9564) (53.2023, 5.9189) (53.037, 5.9176) knots 0.00002 0.00002 0.00002 0.00002 1 1 1 1
  line L245 (53.037, 5.9176) -> (52.3678, 5.9123)
  line L246 (52.3678, 5.9123) -> (52.3889, 3.2553)
  spline S651 degree 3 poles (52.3889, 3.2553) (52.3904, 3.061) (52.3488, 2.8833) (52.23, 2.7523) knots 0 0 0 0 1 1 1 1
  spline S652 degree 3 poles (52.23, 2.7523) (52.1219, 2.6331) (51.9619, 2.5663) (51.8, 2.565) knots 0 0 0 0 1 1 1 1
  spline S653 degree 3 poles (51.8, 2.565) (51.6365, 2.5637) (51.4741, 2.6282) (51.3631, 2.7467) knots 0 0 0 0 1 1 1 1
  spline S654 degree 3 poles (51.3631, 2.7467) (51.2423, 2.8756) (51.1964, 3.0526) (51.1948, 3.2458) knots 0.000017 0.000017 0.000017 0.000017 1 1 1 1
  line L247 (51.1948, 3.2458) -> (51.1737, 5.9028)
  line L248 (51.1737, 5.9028) -> (50.5045, 5.8975)
  spline S655 degree 3 poles (50.5045, 5.8975) (50.3392, 5.8962) (50.1835, 5.9309) (50.066, 6.0357) knots 0 0 0 0 1 1 1 1
  spline S656 degree 3 poles (50.066, 6.0357) (49.9587, 6.1313) (49.8991, 6.2768) (49.8979, 6.42) knots 0.000022 0.000022 0.000022 0.000022 1 1 1 1
  spline S657 degree 3 poles (49.8979, 6.42) (49.8968, 6.567) (49.9567, 6.7177) (50.068, 6.8147) knots 0 0 0 0 1 1 1 1
  spline S658 degree 3 poles (50.068, 6.8147) (50.1834, 6.9153) (50.3354, 6.9535) (50.4961, 6.9548) knots 0.00002 0.00002 0.00002 0.00002 1 1 1 1
  line L249 (50.4961, 6.9548) -> (53.0286, 6.9749)
  spline S659 degree 3 poles (53.0286, 6.9749) (53.1957, 6.9762) (53.3528, 6.941) (53.4712, 6.8353) knots 0 0 0 0 1 1 1 1
  dimension "d1" = 60
  dimension "d2" = 35
  dimension "d3" = 5
  dimension "d4" = 11
  dimension "d5" = 1
  dimension "d7" = 6
  dimension "d8" = 8
  dimension "d20" = 0.2
  dimension "d21" = 0.2
  dimension "d22" = 0.2
  dimension "d29" = 0.2
  dimension "d30" = -0.2
  dimension "d31" = -0.2
  dimension "d32" = -0.2
  dimension "d33" = -0.2
  dimension "d34" = -0.2
  dimension "d35" = -0.2
  dimension "d36" = -0.2
  dimension "d37" = -0.2
  dimension "d38" = -0.2
  dimension "d39" = -0.2
  dimension "d40" = -0.2
  dimension "d41" = -0.2
  dimension "d42" = -0.2
  dimension "d43" = -0.2
  dimension "d44" = -0.2
  dimension "d45" = -0.2
  dimension "d46" = -0.2
  dimension "d47" = -0.2
  dimension "d48" = -0.2
  constraint horizontal L0
  constraint vertical L1
  constraint horizontal L2
  constraint vertical L3
  constraint coincident L0.start L3.end
  constraint vertical L4
  constraint tangent L4 A1
  constraint tangent L5 A1
  constraint vertical L5
  constraint equal L4 L5
  constraint concentric A2 A3
  measures "d1" distance of L0.start L0.end
  measures "d2" distance of L0.start L2.end
  measures "d3" diameter of A0
  measures "d4" diameter of A3
  measures "d5" radius of A1
  measures "d7" distance of L4.start L4.end
  measures "d8" diameter of A2
extrude "Estrusione5" add sketch "Schizzo1" along normal blind 2 contours L0 L1 L2 L3
extrude "Estrusione2" [suppressed]
extrude "Estrusione3" [suppressed]
extrude "Estrusione4" [suppressed]
extrude "Estrusione1" [suppressed]
